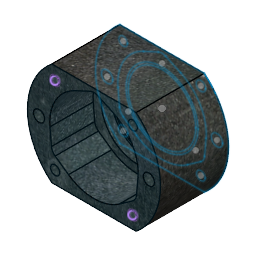
ER25 socket pocket v1 (Autodesk Fusion 360 design; units mm, degrees)
part number: 2026-08-19-05-41-19-233
Autodesk Fusion 360 part; units mm, degrees
sketch "Sketch1" plane through (0, 0, 38.5) normal (0, 0, 1) x (1, 0, 0)
  line L0 (-140.4579, 78.609) -> (-132.0886, 82.4802)
  arc A0 (-127.9114, 82.4802) -> (-132.0886, 82.4802) centre (-130, 77.9648) ccw
  line L1 (-127.9114, 82.4802) -> (-119.5421, 78.609)
  arc A1 (-105.1911, 53.7523) -> (-119.5421, 78.609) centre (-130, 56) ccw
  line L2 (-105.1911, 53.7523) -> (-106.0232, 44.5687)
  arc A2 (-108.1118, 40.9511) -> (-106.0232, 44.5687) centre (-110.9779, 45.0176) ccw
  line L3 (-108.1118, 40.9511) -> (-115.649, 35.6388)
  arc A3 (-144.351, 35.6388) -> (-115.649, 35.6388) centre (-130, 56) ccw
  line L4 (-144.351, 35.6388) -> (-151.8882, 40.9511)
  arc A4 (-153.9768, 44.5687) -> (-151.8882, 40.9511) centre (-149.0221, 45.0176) ccw
  line L5 (-153.9768, 44.5687) -> (-154.8089, 53.7523)
  arc A5 (-140.4579, 78.609) -> (-154.8089, 53.7523) centre (-130, 56) ccw
  circle A6 centre (-108.0914, 34.0914) radius 2.35
  circle A7 centre (-99.0165, 56) radius 3.175
  circle A8 centre (-160.9835, 56) radius 3.175
  circle A9 centre (-151.9086, 77.9086) radius 2.35
  arc A10 (-153.775, 85) -> (-153.775, 27) centre (-130, 56) ccw
  line L6 (-153.775, 27) -> (-106.225, 27)
  arc A11 (-106.225, 27) -> (-106.225, 85) centre (-130, 56) ccw
  line L7 (-106.225, 85) -> (-153.775, 85)
  circle A12 centre (-151.9092, 34.0916) radius 2.6
  circle A13 centre (-108.0914, 77.9086) radius 2.6
  circle A14 centre (-130, 56) radius 19
  circle A15 centre (-130, 56) radius 20.25
  dimension "d3" = 38
  dimension "d4" = 40.5
  dimension "d11" = 4.7
  dimension "d12" = 4.7
  dimension "d15" = 5.2
  dimension "d18" = 5.2
  dimension "d19" = 6.35
  dimension "d20" = 6.35
  constraint concentric A1 A14
  constraint concentric A14 A15
  measures "d3" diameter of A14
  measures "d4" diameter of A15
  measures "d11" diameter of A6
  measures "d12" diameter of A9
  measures "d15" diameter of A12
  measures "d18" diameter of A13
  measures "d19" diameter of A7
  measures "d20" diameter of A8
extrude "Extrude4" add sketch "Sketch1" along normal blind 14 contours L0 A0 L1 A1 L2 A2 L3 A3 L4 A4 L5 A5
extrude "Extrude5" add sketch "Sketch1" along normal blind 8.5 contours A15
extrude "Extrude6" add sketch "Sketch1" along normal blind 38.4 contours A6 | A9 | A10 L6 A11 L7
sketch "Sketch2" plane through (0, 0, 76.9) normal (0, 0, 1) x (1, 0, 0)
  circle A0 centre (-108.0914, 77.9086) radius 2.6
  circle A1 centre (-99.0165, 56) radius 3.175
  circle A2 centre (-151.9092, 34.0916) radius 2.6
  circle A3 centre (-160.9835, 56) radius 3.175
  arc A4 (-127.9114, 82.4802) -> (-132.0886, 82.4802) centre (-130, 77.9648) ccw
  line L0 (-127.9114, 82.4802) -> (-119.5421, 78.609)
  arc A5 (-105.1911, 53.7523) -> (-119.5421, 78.609) centre (-130, 56) ccw
  line L1 (-105.1911, 53.7523) -> (-106.0232, 44.5687)
  arc A6 (-108.1118, 40.9511) -> (-106.0232, 44.5687) centre (-110.9779, 45.0176) ccw
  line L2 (-108.1118, 40.9511) -> (-115.649, 35.6388)
  arc A7 (-144.351, 35.6388) -> (-115.649, 35.6388) centre (-130, 56) ccw
  line L3 (-144.351, 35.6388) -> (-151.8882, 40.9511)
  arc A8 (-153.9768, 44.5687) -> (-151.8882, 40.9511) centre (-149.0221, 45.0176) ccw
  line L4 (-153.9768, 44.5687) -> (-154.8089, 53.7523)
  arc A9 (-140.4579, 78.609) -> (-154.8089, 53.7523) centre (-130, 56) ccw
  line L5 (-140.4579, 78.609) -> (-132.0886, 82.4802)
  line L6 (-106.225, 85) -> (-153.775, 85)
  arc A10 (-153.775, 85) -> (-153.775, 27) centre (-130, 56) ccw
  line L7 (-153.775, 27) -> (-106.225, 27)
  arc A11 (-106.225, 27) -> (-106.225, 85) centre (-130, 56) ccw
  circle A12 centre (-108.0914, 34.0914) radius 2.35
  circle A13 centre (-151.9086, 77.9086) radius 2.35
extrude "Extrude7" cut sketch "Sketch2" against normal blind 7 contours A12 | A13
